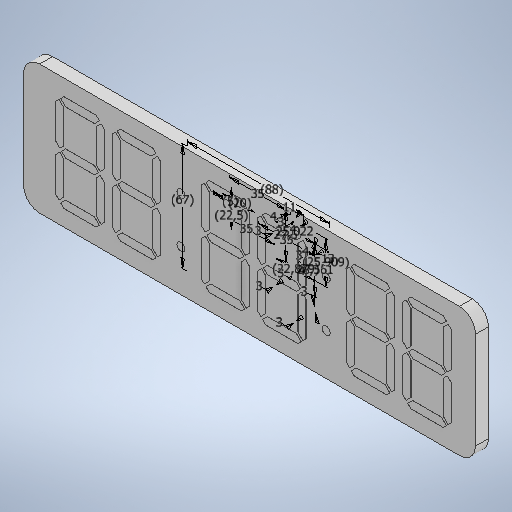
# Autodesk Inventor part: led 7 seg with sec v3
Saved by Autodesk Inventor 2026 (Build 300175000, 175)
## iProperties
Created: 2025-05-20
Part Number: led 7 seg with sec v3
Material: Generic
Document SubType Name: Modeling
Designer: Korobeynikov
Density: 1 g/cm^3
Appearance: Default
Author: Korobeynikov
Autodesk Inventor part; units mm, degrees
(part 1 of 2)
ref_plane "YZ Plane" through (0, 0, 0) normal (1, 0, 0) x (0, 1, 0)
ref_plane "XZ Plane" through (0, 0, 0) normal (0, 1, 0) x (-1, 0, 0)
ref_plane "XY Plane" through (0, 0, 0) normal (0, 0, 1) x (1, 0, 0)
sketch "Sketch1" plane through (0, 0, 0) normal (0, 0, 1) x (1, 0, 0)
  line L0 (-94.452745, 39.06468) -> (-94.589791, 54.989395)
  line L1 (-94.589791, 54.989395) -> (-92.917833, 56.661352)
  line L2 (-92.917833, 56.661352) -> (-89.738372, 53.618937)
  line L3 (-89.738372, 53.618937) -> (-89.519936, 39.107131)
  line L4 (-89.519936, 39.107131) -> (-91.876285, 36.652675)
  line L5 (-91.876285, 36.652675) -> (-94.452745, 39.06468)
  line L6 (-91.726744, 57.81642) -> (-89.962706, 59.534036)
  line L7 (-89.962706, 59.534036) -> (-75.989669, 59.62688)
  line L8 (-75.989669, 59.62688) -> (-74.318475, 57.81642)
  line L9 (-74.318475, 57.81642) -> (-77.243064, 54.845409)
  line L10 (-77.243064, 54.845409) -> (-88.659704, 54.666486)
  line L11 (-88.659704, 54.666486) -> (-91.726744, 57.81642)
  line L12 (-76.216901, 53.807549) -> (-73.431578, 57.037508)
  line L13 (-73.431578, 57.037508) -> (-71.760384, 55.412736)
  line L14 (-71.760384, 55.412736) -> (-71.161775, 39.572555)
  line L15 (-71.161775, 39.572555) -> (-73.390034, 36.97292)
  line L16 (-73.390034, 36.97292) -> (-75.989669, 39.386867)
  line L17 (-75.989669, 39.386867) -> (-76.216901, 53.807549)
  line L18 (-94.41637, 31.993238) -> (-91.950969, 34.351448)
  line L19 (-91.950969, 34.351448) -> (-89.414107, 31.993238)
  line L20 (-89.414107, 31.993238) -> (-89.235455, 17.272291)
  line L21 (-89.235455, 17.272291) -> (-92.344004, 14.02082)
  line L22 (-92.344004, 14.02082) -> (-94.41637, 15.55723)
  line L23 (-94.41637, 15.55723) -> (-94.41637, 31.993238)
  line L24 (-75.729343, 32.350542) -> (-73.442594, 34.780213)
  line L25 (-73.442594, 34.780213) -> (-71.120115, 32.350542)
  line L26 (-71.120115, 32.350542) -> (-70.584158, 16.450491)
  line L27 (-70.584158, 16.450491) -> (-72.227759, 14.449586)
  line L28 (-72.227759, 14.449586) -> (-75.47923, 17.558135)
  line L29 (-75.47923, 17.558135) -> (-75.729343, 32.350542)
  line L30 (-91.320001, 13.041828) -> (-88.199271, 16.093186)
  line L31 (-88.199271, 16.093186) -> (-76.586874, 16.486221)
  line L32 (-76.586874, 16.486221) -> (-73.478325, 13.377672)
  line L33 (-73.478325, 13.377672) -> (-75.014734, 11.62688)
  line L34 (-75.014734, 11.62688) -> (-89.360478, 11.037757)
  line L35 (-89.360478, 11.037757) -> (-91.320001, 13.041828)
  line L36 (-120.187024, 34.985074) -> (-117.790265, 37.349445)
  line L37 (-117.790265, 37.349445) -> (-105.903635, 37.640942)
  line L38 (-105.903635, 37.640942) -> (-103.442099, 35.30896)
  line L39 (-103.442099, 35.30896) -> (-106.000801, 32.847424)
  line L40 (-106.000801, 32.847424) -> (-117.806898, 32.572344)
  line L41 (-117.806898, 32.572344) -> (-120.187024, 34.985074)
  line L42 (-90.850509, 35.606243) -> (-88.45375, 37.970613)
  line L43 (-88.45375, 37.970613) -> (-76.56712, 38.262111)
  line L44 (-76.56712, 38.262111) -> (-74.105584, 35.930129)
  line L45 (-74.105584, 35.930129) -> (-76.664286, 33.468593)
  line L46 (-76.664286, 33.468593) -> (-88.470383, 33.193513)
  line L47 (-88.470383, 33.193513) -> (-90.850509, 35.606243)
  line L48 (-15, -30) -> (15, -30)
  line L49 (15, -30) -> (15, 30)
  line L50 (15, 30) -> (-15, 30)
  line L51 (-15, 30) -> (-15, -30)
  line L52 (-10, 30) -> (-10, -30)
  line L53 (10, 30) -> (10, -30)
  line L54 (-15, 25) -> (15, 25)
  line L55 (-15, -25) -> (15, -25)
  line L56 (-15, 2.5) -> (15, 2.5)
  line L57 (-15, -2.5) -> (15, -2.5)
  circle A0 centre (-12.5, 0) radius 1.06066
  line L58 (-11.43934, 0) -> (-8.93934, 2.5)
  line L59 (-11.43934, 0) -> (-8.93934, -2.5)
  line L60 (-12.5, 1.06066) -> (-15, 3.56066)
  line L61 (-12.5, 1.06066) -> (-10, 3.56066)
  line L62 (-12.5, -1.06066) -> (-15, -3.56066)
  line L63 (-12.5, -1.06066) -> (-10, -3.56066)
  line L64 (0, 8.520255) -> (0, -8.520255)
  line L65 (11.43934, 0) -> (8.93934, 2.5)
  line L66 (11.43934, 0) -> (8.93934, -2.5)
  line L67 (12.5, 1.06066) -> (15, 3.56066)
  line L68 (12.5, 1.06066) -> (10, 3.56066)
  line L69 (12.5, -1.06066) -> (15, -3.56066)
  line L70 (12.5, -1.06066) -> (10, -3.56066)
  line L71 (-15, 25) -> (-10, 30)
  line L72 (-15, 30) -> (-10, 25)
  line L73 (-13.03033, 26.96967) -> (-10, 23.93934)
  line L74 (-11.96967, 28.03033) -> (-8.93934, 25)
  line L75 (-6.230805, 0) -> (6.230805, 0)
  line L76 (13.03033, 26.96967) -> (10, 23.93934)
  line L77 (11.96967, 28.03033) -> (8.93934, 25)
  line L78 (-13.03033, -26.96967) -> (-10, -23.93934)
  line L79 (-11.96967, -28.03033) -> (-8.93934, -25)
  line L80 (13.03033, -26.96967) -> (10, -23.93934)
  line L81 (11.96967, -28.03033) -> (8.93934, -25)
  line L82 (10, 30) -> (15, 25)
  line L83 (-15, -25) -> (-10, -30)
  line L84 (10, -30) -> (15, -25)
  point P0 (0, 0)
  point P1 (-15, 0)
  point P2 (15, 0)
  point P3 (0, 0)
  dimension "d19" = 4.78147
  dimension "d20" = 48.49628
  dimension "d21" = 1.50362
  dimension "d22" = 20.00868
  dimension "d23" = 17.40827
  dimension "d24" = 22.82941
  dimension "d25" = 26.15829
  dimension "d26" = 4.82789
  dimension "d27" = 30
  dimension "d28" = 60
  dimension "d29" = 5
  dimension "d30" = 5
  dimension "d31" = 5
  dimension "d32" = 5
  dimension "d33" = 2.5
  dimension "d34" = 2.5
  dimension "d37" = 2.5
  dimension "d39" = 45
  dimension "d40" = 45
  dimension "d41" = 45
  dimension "d42" = 45
  dimension "d43" = 1.5
  dimension "d44" = 45
  dimension "d47" = 1.67119
  dimension "d50" = 0.75
  dimension "d51" = 0.75
  constraints: 168 end point, 21 symmetric about line, 17 point on line, 11 perpendicular, 3 horizontal alignment, 3 midpoint, 3 parallel, 3 point on circle, 2 horizontal, 2 vertical, 2 vertical alignment, 1 centre point, 1 coincident, 10 other
  measures "d19" vertical distance of L7.end L9.end
  measures "d20" vertical distance of L34.end L6.end
  measures "d21" distance of L10.end L2.end
  measures "d22" vertical distance of L4.end L1.end
  measures "d23" distance of L8.end L6.start
  measures "d24" horizontal distance of L13.end L0.end
  measures "d25" vertical distance of L7.end L45.end
  measures "d26" horizontal distance of L14.end L16.end
  measures "d27" distance of L50.end L49.end
  measures "d28" distance of L49.end L48.end
  measures "d30" distance between parallel lines of L49 L53
  measures "d31" distance between parallel lines of L50 L54
  measures "d32" distance between parallel lines of L48 L55
  measures "d33" distance from line of point (0, 0) L57
  measures "d34" distance from line of point (0, 0) L56
  measures "d37" distance of point (-15, 0) A0.centre
  measures "d39" angle of L57 L59
  measures "d40" angle of L56 L58
  measures "d41" angle to the sketch x axis of L60
  measures "d42" angle of L52 L61
  measures "d43" distance of L58.end L61.end
  measures "d44" angle to the sketch x axis of L62
  measures "d47" horizontal distance of L13.end L12.end
  measures "d50" distance between parallel lines of L72 L73
  measures "d51" distance between parallel lines of L74 L72
extrude "Extrusion1" add sketch "Sketch1" along normal blind 0.5 contours L52 L79 L55 L81 L53 L48 | L83 L79 L52 | L51 L62 L57 L63 L52 L78 L55 | L55 L78 L83 | L53 L81 L84 | L62 L63 L57 | L55 L80 L53 L70 L57 L69 L49 | L84 L80 L55 | L51 L54 L73 L52 L61 L56 L60 | L56 L61 L60 | L58 L52 L59 | L57 L70 L69 | L71 L73 L54 | L52 L58 L56 L64 L57 L59 | L64 L56 L65 L53 L66 L57 | L67 L56 L68 L53 L76 L54 L49 | L67 L68 L56 | L53 L65 L66 | L50 L53 L77 L54 L74 L52 | L52 L74 L71 | L54 L76 L82 | L82 L77 L53
pattern_linear "Rectangular Pattern1" count 2 spacing -35 along (-1, 0, 0) of "Extrusion1"
pattern_linear "Rectangular Pattern2" count 3 spacing 90 along (1, 0, 0) of "Extrusion1", "Rectangular Pattern1"
sketch "Sketch2" plane through (50, 3.56066, 0) normal (0, 0, -1) x (-1, 0, 0)
  line L0 (-25, 21.43934) -> (-25, 0)
  line L1 (-25, 10.71967) -> (0, 10.71967)
  line L2 (0, 0) -> (0, 21.43934)
  line L3 (-25, -7.12132) -> (-25, -28.56066)
  line L4 (-25, -17.84099) -> (0, -17.84099)
  line L5 (0, -28.56066) -> (0, -7.12132)
  circle A0 centre (-12.5, 10.71967) radius 2.5
  circle A1 centre (-12.5, -17.84099) radius 2.5
  line L6 (-115, 21.43934) -> (-115, 0)
  line L7 (-115, 10.71967) -> (-90, 10.71967)
  line L8 (-90, 0) -> (-90, 21.43934)
  line L9 (-115, -7.12132) -> (-115, -28.56066)
  line L10 (-115, -17.84099) -> (-90, -17.84099)
  line L11 (-90, -28.56066) -> (-90, -7.12132)
  circle A2 centre (-102.5, 10.71967) radius 2.5
  circle A3 centre (-102.5, -17.84099) radius 2.5
  point P0 (50, -3.56066)
  dimension "d58" = 5
  dimension "d59" = 5
  dimension "d62" = 12.5
  dimension "d203" = 5
  dimension "d204" = 5
  constraints: 12 midpoint, 8 end point, 4 centre point
  measures "d58" diameter of A0
  measures "d59" diameter of A1
  measures "d62" distance from line of L2 A0.centre
  measures "d203" diameter of A2
  measures "d204" diameter of A3
extrude "Extrusion2" add sketch "Sketch2" against normal up to surface (0.5 mm away)
sketch "Sketch3" plane through (115, 30, 0.5) normal (0, 0, 1) x (1, 0, 0)
  line L0 (-140, 10) -> (120, 10)
  line L1 (130, 0) -> (130, -60)
  line L2 (120, -70) -> (-140, -70)
  line L3 (-150, -60) -> (-150, 0)
  line L4 (25, -26.43934) -> (25, -5)
  line L5 (-130, -5) -> (-130, -26.43934)
  line L6 (-105, 0) -> (-125, 0)
  line L7 (-125, -60) -> (-105, -60)
  arc A0 (-140, 10) -> (-150, 0) centre (-140, 0) ccw
  arc A1 (-150, -60) -> (-140, -70) centre (-140, -60) ccw
  arc A2 (130, 0) -> (120, 10) centre (120, 0) ccw
  arc A3 (120, -70) -> (130, -60) centre (120, -60) ccw
  line L8 (-103.03033, -1.96967) -> (-105, 0)
  line L9 (-105, 0) -> (-125, 0)
  line L10 (-125, 0) -> (-126.96967, -1.96967)
  line L11 (-126.96967, -1.96967) -> (-123.93934, -5)
  line L12 (-123.93934, -5) -> (-106.06066, -5)
  line L13 (-106.06066, -5) -> (-103.03033, -1.96967)
  line L14 (-128.03033, -3.03033) -> (-130, -5)
  line L15 (-130, -5) -> (-130, -26.43934)
  line L16 (-130, -26.43934) -> (-127.5, -28.93934)
  line L17 (-127.5, -28.93934) -> (-125, -26.43934)
  line L18 (-125, -26.43934) -> (-125, -6.06066)
  line L19 (-125, -6.06066) -> (-128.03033, -3.03033)
  line L20 (-123.93934, -27.5) -> (-126.43934, -30)
  line L21 (-126.43934, -30) -> (-123.93934, -32.5)
  line L22 (-123.93934, -32.5) -> (-106.06066, -32.5)
  line L23 (-106.06066, -32.5) -> (-103.56066, -30)
  line L24 (-103.56066, -30) -> (-106.06066, -27.5)
  line L25 (-106.06066, -27.5) -> (-123.93934, -27.5)
  line L26 (-125, -53.93934) -> (-125, -33.56066)
  line L27 (-130, -33.56066) -> (-130, -55)
  line L28 (-125, -53.93934) -> (-125, -33.56066)
  line L29 (-125, -33.56066) -> (-127.5, -31.06066)
  line L30 (-127.5, -31.06066) -> (-130, -33.56066)
  line L31 (-130, -33.56066) -> (-130, -55)
  line L32 (-130, -55) -> (-128.03033, -56.96967)
  line L33 (-128.03033, -56.96967) -> (-125, -53.93934)
  line L34 (-106.06066, -55) -> (-123.93934, -55)
  line L35 (-106.06066, -55) -> (-123.93934, -55)
  line L36 (-123.93934, -55) -> (-126.96967, -58.03033)
  line L37 (-126.96967, -58.03033) -> (-125, -60)
  line L38 (-125, -60) -> (-105, -60)
  line L39 (-105, -60) -> (-103.03033, -58.03033)
  line L40 (-103.03033, -58.03033) -> (-106.06066, -55)
  line L41 (-101.96967, -56.96967) -> (-100, -55)
  line L42 (-100, -55) -> (-100, -33.56066)
  line L43 (-100, -33.56066) -> (-102.5, -31.06066)
  line L44 (-102.5, -31.06066) -> (-105, -33.56066)
  line L45 (-105, -33.56066) -> (-105, -53.93934)
  line L46 (-105, -53.93934) -> (-101.96967, -56.96967)
  line L47 (-105, -6.06066) -> (-105, -26.43934)
  line L48 (-105, -26.43934) -> (-102.5, -28.93934)
  line L49 (-102.5, -28.93934) -> (-100, -26.43934)
  line L50 (-100, -26.43934) -> (-100, -5)
  line L51 (-100, -5) -> (-101.96967, -3.03033)
  line L52 (-101.96967, -3.03033) -> (-105, -6.06066)
  line L53 (-90, -26.43934) -> (-90, -6.06066)
  line L54 (-93.03033, -3.03033) -> (-95, -5)
  line L55 (-95, -5) -> (-95, -26.43934)
  line L56 (-95, -26.43934) -> (-92.5, -28.93934)
  line L57 (-92.5, -28.93934) -> (-90, -26.43934)
  line L58 (-90, -26.43934) -> (-90, -6.06066)
  line L59 (-90, -6.06066) -> (-93.03033, -3.03033)
  line L60 (-68.03033, -1.96967) -> (-70, 0)
  line L61 (-70, 0) -> (-90, 0)
  line L62 (-90, 0) -> (-91.96967, -1.96967)
  line L63 (-91.96967, -1.96967) -> (-88.93934, -5)
  line L64 (-88.93934, -5) -> (-71.06066, -5)
  line L65 (-71.06066, -5) -> (-68.03033, -1.96967)
  line L66 (-70, -6.06066) -> (-70, -26.43934)
  line L67 (-70, -26.43934) -> (-67.5, -28.93934)
  line L68 (-67.5, -28.93934) -> (-65, -26.43934)
  line L69 (-65, -26.43934) -> (-65, -5)
  line L70 (-65, -5) -> (-66.96967, -3.03033)
  line L71 (-66.96967, -3.03033) -> (-70, -6.06066)
  line L72 (-88.93934, -27.5) -> (-91.43934, -30)
  line L73 (-91.43934, -30) -> (-88.93934, -32.5)
  line L74 (-88.93934, -32.5) -> (-71.06066, -32.5)
  line L75 (-71.06066, -32.5) -> (-68.56066, -30)
  line L76 (-68.56066, -30) -> (-71.06066, -27.5)
  line L77 (-71.06066, -27.5) -> (-88.93934, -27.5)
  line L78 (-95, -33.56066) -> (-95, -55)
  line L79 (-90, -53.93934) -> (-90, -33.56066)
  line L80 (-90, -33.56066) -> (-92.5, -31.06066)
  line L81 (-92.5, -31.06066) -> (-95, -33.56066)
  line L82 (-95, -33.56066) -> (-95, -55)
  line L83 (-95, -55) -> (-93.03033, -56.96967)
  line L84 (-93.03033, -56.96967) -> (-90, -53.93934)
  line L85 (-66.96967, -56.96967) -> (-65, -55)
  line L86 (-65, -55) -> (-65, -33.56066)
  line L87 (-65, -33.56066) -> (-67.5, -31.06066)
  line L88 (-67.5, -31.06066) -> (-70, -33.56066)
  line L89 (-70, -33.56066) -> (-70, -53.93934)
  line L90 (-70, -53.93934) -> (-66.96967, -56.96967)
  line L91 (-71.06066, -55) -> (-88.93934, -55)
  line L92 (-88.93934, -55) -> (-91.96967, -58.03033)
  line L93 (-91.96967, -58.03033) -> (-90, -60)
  line L94 (-90, -60) -> (-70, -60)
  line L95 (-70, -60) -> (-68.03033, -58.03033)
  line L96 (-68.03033, -58.03033) -> (-71.06066, -55)
  circle A4 centre (-52.5, -44.28033) radius 2.5
  circle A5 centre (-52.5, -15.71967) radius 2.5
  line L97 (-40, -5) -> (-40, -26.43934)
  line L98 (-13.03033, -1.96967) -> (-15, 0)
  line L99 (-15, 0) -> (-35, 0)
  line L100 (-35, 0) -> (-36.96967, -1.96967)
  line L101 (-36.96967, -1.96967) -> (-33.93934, -5)
  line L102 (-33.93934, -5) -> (-16.06066, -5)
  line L103 (-16.06066, -5) -> (-13.03033, -1.96967)
  line L104 (-15, -6.06066) -> (-15, -26.43934)
  line L105 (-15, -26.43934) -> (-12.5, -28.93934)
  line L106 (-12.5, -28.93934) -> (-10, -26.43934)
  line L107 (-10, -26.43934) -> (-10, -5)
  line L108 (-10, -5) -> (-11.96967, -3.03033)
  line L109 (-11.96967, -3.03033) -> (-15, -6.06066)
  line L110 (-38.03033, -3.03033) -> (-40, -5)
  line L111 (-40, -5) -> (-40, -26.43934)
  line L112 (-40, -26.43934) -> (-37.5, -28.93934)
  line L113 (-37.5, -28.93934) -> (-35, -26.43934)
  line L114 (-35, -26.43934) -> (-35, -6.06066)
  line L115 (-35, -6.06066) -> (-38.03033, -3.03033)
  line L116 (-33.93934, -27.5) -> (-36.43934, -30)
  line L117 (-36.43934, -30) -> (-33.93934, -32.5)
  line L118 (-33.93934, -32.5) -> (-16.06066, -32.5)
  line L119 (-16.06066, -32.5) -> (-13.56066, -30)
  line L120 (-13.56066, -30) -> (-16.06066, -27.5)
  line L121 (-16.06066, -27.5) -> (-33.93934, -27.5)
  line L122 (-35, -53.93934) -> (-35, -33.56066)
  line L123 (-35, -33.56066) -> (-37.5, -31.06066)
  line L124 (-37.5, -31.06066) -> (-40, -33.56066)
  line L125 (-40, -33.56066) -> (-40, -55)
  line L126 (-40, -55) -> (-38.03033, -56.96967)
  line L127 (-38.03033, -56.96967) -> (-35, -53.93934)
  line L128 (-16.06066, -55) -> (-33.93934, -55)
  line L129 (-33.93934, -55) -> (-36.96967, -58.03033)
  line L130 (-36.96967, -58.03033) -> (-35, -60)
  line L131 (-35, -60) -> (-15, -60)
  line L132 (-15, -60) -> (-13.03033, -58.03033)
  line L133 (-13.03033, -58.03033) -> (-16.06066, -55)
  line L134 (-11.96967, -56.96967) -> (-10, -55)
  line L135 (-10, -55) -> (-10, -33.56066)
  line L136 (-10, -33.56066) -> (-12.5, -31.06066)
  line L137 (-12.5, -31.06066) -> (-15, -33.56066)
  line L138 (-15, -33.56066) -> (-15, -53.93934)
  line L139 (-15, -53.93934) -> (-11.96967, -56.96967)
  line L140 (0, -53.93934) -> (0, -33.56066)
  line L141 (0, -33.56066) -> (-2.5, -31.06066)
  line L142 (-2.5, -31.06066) -> (-5, -33.56066)
  line L143 (-5, -33.56066) -> (-5, -55)
  line L144 (-5, -55) -> (-3.03033, -56.96967)
  line L145 (-3.03033, -56.96967) -> (0, -53.93934)
  line L146 (1.06066, -27.5) -> (-1.43934, -30)
  line L147 (-1.43934, -30) -> (1.06066, -32.5)
  line L148 (1.06066, -32.5) -> (18.93934, -32.5)
  line L149 (18.93934, -32.5) -> (21.43934, -30)
  line L150 (21.43934, -30) -> (18.93934, -27.5)
  line L151 (18.93934, -27.5) -> (1.06066, -27.5)
  line L152 (-3.03033, -3.03033) -> (-5, -5)
  line L153 (-5, -5) -> (-5, -26.43934)
  line L154 (-5, -26.43934) -> (-2.5, -28.93934)
  line L155 (-2.5, -28.93934) -> (0, -26.43934)
  line L156 (0, -26.43934) -> (0, -6.06066)
  line L157 (0, -6.06066) -> (-3.03033, -3.03033)
  line L158 (21.96967, -1.96967) -> (20, 0)
  line L159 (20, 0) -> (0, 0)
  line L160 (0, 0) -> (-1.96967, -1.96967)
  line L161 (-1.96967, -1.96967) -> (1.06066, -5)
  line L162 (1.06066, -5) -> (18.93934, -5)
  line L163 (18.93934, -5) -> (21.96967, -1.96967)
  line L164 (20, -6.06066) -> (20, -26.43934)
  line L165 (20, -26.43934) -> (22.5, -28.93934)
  line L166 (22.5, -28.93934) -> (25, -26.43934)
  line L167 (25, -26.43934) -> (25, -5)
  line L168 (25, -5) -> (23.03033, -3.03033)
  line L169 (23.03033, -3.03033) -> (20, -6.06066)
  line L170 (23.03033, -56.96967) -> (25, -55)
  line L171 (25, -55) -> (25, -33.56066)
  line L172 (25, -33.56066) -> (22.5, -31.06066)
  line L173 (22.5, -31.06066) -> (20, -33.56066)
  line L174 (20, -33.56066) -> (20, -53.93934)
  line L175 (20, -53.93934) -> (23.03033, -56.96967)
  line L176 (18.93934, -55) -> (1.06066, -55)
  line L177 (1.06066, -55) -> (-1.96967, -58.03033)
  line L178 (-1.96967, -58.03033) -> (0, -60)
  line L179 (0, -60) -> (20, -60)
  line L180 (20, -60) -> (21.96967, -58.03033)
  line L181 (21.96967, -58.03033) -> (18.93934, -55)
  line L182 (115, -26.43934) -> (115, -5)
  line L183 (111.96967, -1.96967) -> (110, 0)
  line L184 (108.93934, -5) -> (111.96967, -1.96967)
  line L185 (91.06066, -5) -> (108.93934, -5)
  line L186 (88.03033, -1.96967) -> (91.06066, -5)
  line L187 (90, 0) -> (88.03033, -1.96967)
  line L188 (110, 0) -> (90, 0)
  line L189 (110, -6.06066) -> (110, -26.43934)
  line L190 (113.03033, -3.03033) -> (110, -6.06066)
  line L191 (115, -5) -> (113.03033, -3.03033)
  line L192 (115, -26.43934) -> (115, -5)
  line L193 (112.5, -28.93934) -> (115, -26.43934)
  line L194 (110, -26.43934) -> (112.5, -28.93934)
  line L195 (113.03033, -56.96967) -> (115, -55)
  line L196 (110, -53.93934) -> (113.03033, -56.96967)
  line L197 (110, -33.56066) -> (110, -53.93934)
  line L198 (112.5, -31.06066) -> (110, -33.56066)
  line L199 (115, -33.56066) -> (112.5, -31.06066)
  line L200 (115, -55) -> (115, -33.56066)
  line L201 (91.06066, -27.5) -> (88.56066, -30)
  line L202 (108.93934, -27.5) -> (91.06066, -27.5)
  line L203 (111.43934, -30) -> (108.93934, -27.5)
  line L204 (108.93934, -32.5) -> (111.43934, -30)
  line L205 (91.06066, -32.5) -> (108.93934, -32.5)
  line L206 (88.56066, -30) -> (91.06066, -32.5)
  line L207 (90, -53.93934) -> (90, -33.56066)
  line L208 (86.96967, -56.96967) -> (90, -53.93934)
  line L209 (85, -55) -> (86.96967, -56.96967)
  line L210 (85, -33.56066) -> (85, -55)
  line L211 (87.5, -31.06066) -> (85, -33.56066)
  line L212 (90, -33.56066) -> (87.5, -31.06066)
  line L213 (108.93934, -55) -> (91.06066, -55)
  line L214 (111.96967, -58.03033) -> (108.93934, -55)
  line L215 (110, -60) -> (111.96967, -58.03033)
  line L216 (90, -60) -> (110, -60)
  line L217 (88.03033, -58.03033) -> (90, -60)
  line L218 (91.06066, -55) -> (88.03033, -58.03033)
  line L219 (86.96967, -3.03033) -> (85, -5)
  line L220 (90, -6.06066) -> (86.96967, -3.03033)
  line L221 (90, -26.43934) -> (90, -6.06066)
  line L222 (87.5, -28.93934) -> (90, -26.43934)
  line L223 (85, -26.43934) -> (87.5, -28.93934)
  line L224 (85, -5) -> (85, -26.43934)
  line L225 (76.96967, -1.96967) -> (75, 0)
  line L226 (73.93934, -5) -> (76.96967, -1.96967)
  line L227 (56.06066, -5) -> (73.93934, -5)
  line L228 (53.03033, -1.96967) -> (56.06066, -5)
  line L229 (55, 0) -> (53.03033, -1.96967)
  line L230 (75, 0) -> (55, 0)
  line L231 (75, -6.06066) -> (75, -26.43934)
  line L232 (78.03033, -3.03033) -> (75, -6.06066)
  line L233 (80, -5) -> (78.03033, -3.03033)
  line L234 (80, -26.43934) -> (80, -5)
  line L235 (77.5, -28.93934) -> (80, -26.43934)
  line L236 (75, -26.43934) -> (77.5, -28.93934)
  line L237 (56.06066, -27.5) -> (53.56066, -30)
  line L238 (73.93934, -27.5) -> (56.06066, -27.5)
  line L239 (76.43934, -30) -> (73.93934, -27.5)
  line L240 (73.93934, -32.5) -> (76.43934, -30)
  line L241 (56.06066, -32.5) -> (73.93934, -32.5)
  line L242 (53.56066, -30) -> (56.06066, -32.5)
  line L243 (78.03033, -56.96967) -> (80, -55)
  line L244 (75, -53.93934) -> (78.03033, -56.96967)
  line L245 (75, -33.56066) -> (75, -53.93934)
  line L246 (77.5, -31.06066) -> (75, -33.56066)
  line L247 (80, -33.56066) -> (77.5, -31.06066)
  line L248 (80, -55) -> (80, -33.56066)
  line L249 (73.93934, -55) -> (56.06066, -55)
  line L250 (76.96967, -58.03033) -> (73.93934, -55)
  line L251 (75, -60) -> (76.96967, -58.03033)
  line L252 (55, -60) -> (75, -60)
  line L253 (53.03033, -58.03033) -> (55, -60)
  line L254 (56.06066, -55) -> (53.03033, -58.03033)
  line L255 (55, -53.93934) -> (55, -33.56066)
  line L256 (51.96967, -56.96967) -> (55, -53.93934)
  line L257 (50, -55) -> (51.96967, -56.96967)
  line L258 (50, -33.56066) -> (50, -55)
  line L259 (52.5, -31.06066) -> (50, -33.56066)
  line L260 (55, -33.56066) -> (52.5, -31.06066)
  line L261 (51.96967, -3.03033) -> (50, -5)
  line L262 (55, -6.06066) -> (51.96967, -3.03033)
  line L263 (55, -26.43934) -> (55, -6.06066)
  line L264 (52.5, -28.93934) -> (55, -26.43934)
  line L265 (50, -26.43934) -> (52.5, -28.93934)
  line L266 (50, -5) -> (50, -26.43934)
  circle A6 centre (37.5, -44.28033) radius 2.5
  circle A7 centre (37.5, -15.71967) radius 2.5
  point P0 (-115, -30)
  dimension "d64" = 20
  dimension "d65" = 10
  dimension "d66" = 10
  dimension "d67" = 10
  dimension "d68" = 10
  dimension "d205" = 15
  dimension "d206" = 280
  constraints: 8 end point, 8 point on circle, 8 tangent, 4 centre point, 2 equal radius, 2 parallel, 1 horizontal, 1 perpendicular
  measures "d64" distance between parallel lines of L3 L5
  measures "d65" distance between parallel lines of L6 L0
  measures "d66" distance between parallel lines of L2 L7
  measures "d67" radius of A0
  measures "d68" radius of A1
  measures "d205" distance between parallel lines of L1 L182
  measures "d206" distance between parallel lines of L3 L1
extrude "Extrusion3" add sketch "Sketch3" along normal blind 0.05 and the other way blind 8
sketch "Sketch4" plane through (115, 30, -7.5) normal (0, 0, -1) x (-1, 0, 0)
  line L0 (-120, -70) -> (140, -70)
  arc A0 (140, -70) -> (150, -60) centre (140, -60) ccw
  line L1 (150, -60) -> (150, 0)
  arc A1 (150, 0) -> (140, 10) centre (140, 0) ccw
  line L2 (140, 10) -> (-120, 10)
  arc A2 (-120, 10) -> (-130, 0) centre (-120, 0) ccw
  line L3 (-130, 0) -> (-130, -60)
  arc A3 (-130, -60) -> (-120, -70) centre (-120, -60) ccw
  circle A4 centre (52.5, -15.71967) radius 2.5
  line L4 (-22.5, -28.93934) -> (-25, -26.43934)
  line L5 (-25, -26.43934) -> (-25, -5)
  line L6 (-25, -5) -> (-23.03033, -3.03033)
  line L7 (-23.03033, -3.03033) -> (-20, -6.06066)
  line L8 (-20, -6.06066) -> (-20, -26.43934)
  line L9 (-20, -26.43934) -> (-22.5, -28.93934)
  line L10 (128.03033, -3.03033) -> (130, -5)
  line L11 (130, -5) -> (130, -26.43934)
  line L12 (130, -26.43934) -> (127.5, -28.93934)
  line L13 (127.5, -28.93934) -> (125, -26.43934)
  line L14 (125, -26.43934) -> (125, -6.06066)
  line L15 (125, -6.06066) -> (128.03033, -3.03033)
  line L16 (103.03033, -1.96967) -> (105, 0)
  line L17 (105, 0) -> (125, 0)
  line L18 (125, 0) -> (126.96967, -1.96967)
  line L19 (126.96967, -1.96967) -> (123.93934, -5)
  line L20 (123.93934, -5) -> (106.06066, -5)
  line L21 (106.06066, -5) -> (103.03033, -1.96967)
  line L22 (126.96967, -58.03033) -> (125, -60)
  line L23 (125, -60) -> (105, -60)
  line L24 (105, -60) -> (103.03033, -58.03033)
  line L25 (103.03033, -58.03033) -> (106.06066, -55)
  line L26 (106.06066, -55) -> (123.93934, -55)
  line L27 (123.93934, -55) -> (126.96967, -58.03033)
  line L28 (127.5, -31.06066) -> (130, -33.56066)
  line L29 (130, -33.56066) -> (130, -55)
  line L30 (130, -55) -> (128.03033, -56.96967)
  line L31 (128.03033, -56.96967) -> (125, -53.93934)
  line L32 (125, -53.93934) -> (125, -33.56066)
  line L33 (125, -33.56066) -> (127.5, -31.06066)
  line L34 (92.5, -28.93934) -> (90, -26.43934)
  line L35 (90, -26.43934) -> (90, -6.06066)
  line L36 (90, -6.06066) -> (93.03033, -3.03033)
  line L37 (93.03033, -3.03033) -> (95, -5)
  line L38 (95, -5) -> (95, -26.43934)
  line L39 (95, -26.43934) -> (92.5, -28.93934)
  line L40 (92.5, -31.06066) -> (95, -33.56066)
  line L41 (95, -33.56066) -> (95, -55)
  line L42 (95, -55) -> (93.03033, -56.96967)
  line L43 (93.03033, -56.96967) -> (90, -53.93934)
  line L44 (90, -53.93934) -> (90, -33.56066)
  line L45 (90, -33.56066) -> (92.5, -31.06066)
  circle A5 centre (52.5, -44.28033) radius 2.5
  line L46 (38.03033, -3.03033) -> (40, -5)
  line L47 (40, -5) -> (40, -26.43934)
  line L48 (40, -26.43934) -> (37.5, -28.93934)
  line L49 (37.5, -28.93934) -> (35, -26.43934)
  line L50 (35, -26.43934) -> (35, -6.06066)
  line L51 (35, -6.06066) -> (38.03033, -3.03033)
  line L52 (-21.96967, -58.03033) -> (-18.93934, -55)
  line L53 (-18.93934, -55) -> (-1.06066, -55)
  line L54 (-1.06066, -55) -> (1.96967, -58.03033)
  line L55 (1.96967, -58.03033) -> (0, -60)
  line L56 (0, -60) -> (-20, -60)
  line L57 (-20, -60) -> (-21.96967, -58.03033)
  line L58 (-20, -53.93934) -> (-23.03033, -56.96967)
  line L59 (-23.03033, -56.96967) -> (-25, -55)
  line L60 (-25, -55) -> (-25, -33.56066)
  line L61 (-25, -33.56066) -> (-22.5, -31.06066)
  line L62 (-22.5, -31.06066) -> (-20, -33.56066)
  line L63 (-20, -33.56066) -> (-20, -53.93934)
  line L64 (-18.93934, -5) -> (-21.96967, -1.96967)
  line L65 (-21.96967, -1.96967) -> (-20, 0)
  line L66 (-20, 0) -> (0, 0)
  line L67 (0, 0) -> (1.96967, -1.96967)
  line L68 (1.96967, -1.96967) -> (-1.06066, -5)
  line L69 (-1.06066, -5) -> (-18.93934, -5)
  line L70 (0, -6.06066) -> (3.03033, -3.03033)
  line L71 (3.03033, -3.03033) -> (5, -5)
  line L72 (5, -5) -> (5, -26.43934)
  line L73 (5, -26.43934) -> (2.5, -28.93934)
  line L74 (2.5, -28.93934) -> (0, -26.43934)
  line L75 (0, -26.43934) -> (0, -6.06066)
  line L76 (-18.93934, -27.5) -> (-1.06066, -27.5)
  line L77 (-1.06066, -27.5) -> (1.43934, -30)
  line L78 (1.43934, -30) -> (-1.06066, -32.5)
  line L79 (-1.06066, -32.5) -> (-18.93934, -32.5)
  line L80 (-18.93934, -32.5) -> (-21.43934, -30)
  line L81 (-21.43934, -30) -> (-18.93934, -27.5)
  line L82 (3.03033, -56.96967) -> (0, -53.93934)
  line L83 (0, -53.93934) -> (0, -33.56066)
  line L84 (0, -33.56066) -> (2.5, -31.06066)
  line L85 (2.5, -31.06066) -> (5, -33.56066)
  line L86 (5, -33.56066) -> (5, -55)
  line L87 (5, -55) -> (3.03033, -56.96967)
  line L88 (15, -53.93934) -> (11.96967, -56.96967)
  line L89 (11.96967, -56.96967) -> (10, -55)
  line L90 (10, -55) -> (10, -33.56066)
  line L91 (10, -33.56066) -> (12.5, -31.06066)
  line L92 (12.5, -31.06066) -> (15, -33.56066)
  line L93 (15, -33.56066) -> (15, -53.93934)
  line L94 (13.03033, -58.03033) -> (16.06066, -55)
  line L95 (16.06066, -55) -> (33.93934, -55)
  line L96 (33.93934, -55) -> (36.96967, -58.03033)
  line L97 (36.96967, -58.03033) -> (35, -60)
  line L98 (35, -60) -> (15, -60)
  line L99 (15, -60) -> (13.03033, -58.03033)
  line L100 (38.03033, -56.96967) -> (35, -53.93934)
  line L101 (35, -53.93934) -> (35, -33.56066)
  line L102 (35, -33.56066) -> (37.5, -31.06066)
  line L103 (37.5, -31.06066) -> (40, -33.56066)
  line L104 (40, -33.56066) -> (40, -55)
  line L105 (40, -55) -> (38.03033, -56.96967)
  line L106 (16.06066, -27.5) -> (33.93934, -27.5)
  line L107 (33.93934, -27.5) -> (36.43934, -30)
  line L108 (36.43934, -30) -> (33.93934, -32.5)
  line L109 (33.93934, -32.5) -> (16.06066, -32.5)
  line L110 (16.06066, -32.5) -> (13.56066, -30)
  line L111 (13.56066, -30) -> (16.06066, -27.5)
  line L112 (11.96967, -3.03033) -> (15, -6.06066)
  line L113 (15, -6.06066) -> (15, -26.43934)
  line L114 (15, -26.43934) -> (12.5, -28.93934)
  line L115 (12.5, -28.93934) -> (10, -26.43934)
  line L116 (10, -26.43934) -> (10, -5)
  line L117 (10, -5) -> (11.96967, -3.03033)
  line L118 (16.06066, -5) -> (13.03033, -1.96967)
  line L119 (13.03033, -1.96967) -> (15, 0)
  line L120 (15, 0) -> (35, 0)
  line L121 (35, 0) -> (36.96967, -1.96967)
  line L122 (36.96967, -1.96967) -> (33.93934, -5)
  line L123 (33.93934, -5) -> (16.06066, -5)
  line L124 (68.03033, -58.03033) -> (71.06066, -55)
  line L125 (71.06066, -55) -> (88.93934, -55)
  line L126 (88.93934, -55) -> (91.96967, -58.03033)
  line L127 (91.96967, -58.03033) -> (90, -60)
  line L128 (90, -60) -> (70, -60)
  line L129 (70, -60) -> (68.03033, -58.03033)
  line L130 (70, -53.93934) -> (66.96967, -56.96967)
  line L131 (66.96967, -56.96967) -> (65, -55)
  line L132 (65, -55) -> (65, -33.56066)
  line L133 (65, -33.56066) -> (67.5, -31.06066)
  line L134 (67.5, -31.06066) -> (70, -33.56066)
  line L135 (70, -33.56066) -> (70, -53.93934)
  line L136 (71.06066, -27.5) -> (88.93934, -27.5)
  line L137 (88.93934, -27.5) -> (91.43934, -30)
  line L138 (91.43934, -30) -> (88.93934, -32.5)
  line L139 (88.93934, -32.5) -> (71.06066, -32.5)
  line L140 (71.06066, -32.5) -> (68.56066, -30)
  line L141 (68.56066, -30) -> (71.06066, -27.5)
  line L142 (66.96967, -3.03033) -> (70, -6.06066)
  line L143 (70, -6.06066) -> (70, -26.43934)
  line L144 (70, -26.43934) -> (67.5, -28.93934)
  line L145 (67.5, -28.93934) -> (65, -26.43934)
  line L146 (65, -26.43934) -> (65, -5)
  line L147 (65, -5) -> (66.96967, -3.03033)
  line L148 (71.06066, -5) -> (68.03033, -1.96967)
  line L149 (68.03033, -1.96967) -> (70, 0)
  line L150 (70, 0) -> (90, 0)
  line L151 (90, 0) -> (91.96967, -1.96967)
  line L152 (91.96967, -1.96967) -> (88.93934, -5)
  line L153 (88.93934, -5) -> (71.06066, -5)
  line L154 (101.96967, -3.03033) -> (105, -6.06066)
  line L155 (105, -6.06066) -> (105, -26.43934)
  line L156 (105, -26.43934) -> (102.5, -28.93934)
  line L157 (102.5, -28.93934) -> (100, -26.43934)
  line L158 (100, -26.43934) -> (100, -5)
  line L159 (100, -5) -> (101.96967, -3.03033)
  line L160 (105, -53.93934) -> (101.96967, -56.96967)
  line L161 (101.96967, -56.96967) -> (100, -55)
  line L162 (100, -55) -> (100, -33.56066)
  line L163 (100, -33.56066) -> (102.5, -31.06066)
  line L164 (102.5, -31.06066) -> (105, -33.56066)
  line L165 (105, -33.56066) -> (105, -53.93934)
  line L166 (106.06066, -27.5) -> (123.93934, -27.5)
  line L167 (123.93934, -27.5) -> (126.43934, -30)
  line L168 (126.43934, -30) -> (123.93934, -32.5)
  line L169 (123.93934, -32.5) -> (106.06066, -32.5)
  line L170 (106.06066, -32.5) -> (103.56066, -30)
  line L171 (103.56066, -30) -> (106.06066, -27.5)
  line L172 (-120, 8) -> (140, 8)
  arc A6 (148, 0) -> (140, 8) centre (140, 0) ccw
  line L173 (148, 0) -> (148, -60)
  arc A7 (140, -68) -> (148, -60) centre (140, -60) ccw
  line L174 (140, -68) -> (-120, -68)
  arc A8 (-128, -60) -> (-120, -68) centre (-120, -60) ccw
  line L175 (-128, -60) -> (-128, 0)
  arc A9 (-120, 8) -> (-128, 0) centre (-120, 0) ccw
  line L176 (-20, -5) -> (0, -5)
  line L177 (0, -5) -> (0, -27.5)
  line L178 (0, -27.5) -> (-20, -27.5)
  line L179 (-20, -27.5) -> (-20, -5)
  line L180 (-20, -32.5) -> (0, -32.5)
  line L181 (0, -32.5) -> (0, -55)
  line L182 (0, -55) -> (-20, -55)
  line L183 (-20, -55) -> (-20, -32.5)
  line L184 (-18.5, -6.5) -> (-1.5, -6.5)
  line L185 (-1.5, -6.5) -> (-1.5, -26)
  line L186 (-1.5, -26) -> (-18.5, -26)
  line L187 (-18.5, -26) -> (-18.5, -6.5)
  line L188 (-1.5, -34) -> (-18.5, -34)
  line L189 (-18.5, -34) -> (-18.5, -53.5)
  line L190 (-18.5, -53.5) -> (-1.5, -53.5)
  line L191 (-1.5, -53.5) -> (-1.5, -34)
  line L192 (16.5, -6.5) -> (33.5, -6.5)
  line L193 (16.5, -26) -> (16.5, -6.5)
  line L194 (33.5, -6.5) -> (33.5, -26)
  line L195 (33.5, -26) -> (16.5, -26)
  line L196 (33.5, -34) -> (16.5, -34)
  line L197 (16.5, -34) -> (16.5, -53.5)
  line L198 (33.5, -53.5) -> (33.5, -34)
  line L199 (16.5, -53.5) -> (33.5, -53.5)
  line L200 (71.5, -26) -> (71.5, -6.5)
  line L201 (71.5, -6.5) -> (88.5, -6.5)
  line L202 (88.5, -6.5) -> (88.5, -26)
  line L203 (88.5, -26) -> (71.5, -26)
  line L204 (88.5, -34) -> (71.5, -34)
  line L205 (71.5, -34) -> (71.5, -53.5)
  line L206 (88.5, -53.5) -> (88.5, -34)
  line L207 (71.5, -53.5) -> (88.5, -53.5)
  line L208 (106.5, -26) -> (106.5, -6.5)
  line L209 (106.5, -6.5) -> (123.5, -6.5)
  line L210 (123.5, -6.5) -> (123.5, -26)
  line L211 (123.5, -26) -> (106.5, -26)
  line L212 (123.5, -34) -> (106.5, -34)
  line L213 (123.5, -53.5) -> (123.5, -34)
  line L214 (106.5, -34) -> (106.5, -53.5)
  line L215 (106.5, -53.5) -> (123.5, -53.5)
  line L216 (-25, 0) -> (40, 0)
  line L217 (40, 0) -> (40, -60)
  line L218 (40, -60) -> (-25, -60)
  line L219 (-25, -60) -> (-25, 0)
  line L220 (41.5, 1.5) -> (-26.5, 1.5)
  line L221 (-26.5, 1.5) -> (-26.5, -61.5)
  line L222 (-26.5, -61.5) -> (41.5, -61.5)
  line L223 (41.5, -61.5) -> (41.5, 1.5)
  line L224 (131.5, 1.5) -> (63.5, 1.5)
  line L225 (63.5, 1.5) -> (63.5, -61.5)
  line L226 (131.5, -61.5) -> (131.5, 1.5)
  line L227 (63.5, -61.5) -> (131.5, -61.5)
  circle A10 centre (52.5, -15.71967) radius 4
  circle A11 centre (52.5, -44.28033) radius 4
  line L228 (-48.5, 1.5) -> (-116.5, 1.5)
  line L229 (-48.5, -61.5) -> (-48.5, 1.5)
  line L230 (-116.5, -61.5) -> (-48.5, -61.5)
  line L231 (-116.5, 1.5) -> (-116.5, -61.5)
  line L232 (-108.5, -26) -> (-108.5, -6.5)
  line L233 (-108.5, -6.5) -> (-91.5, -6.5)
  line L234 (-91.5, -6.5) -> (-91.5, -26)
  line L235 (-91.5, -26) -> (-108.5, -26)
  line L236 (-91.5, -34) -> (-108.5, -34)
  line L237 (-108.5, -34) -> (-108.5, -53.5)
  line L238 (-108.5, -53.5) -> (-91.5, -53.5)
  line L239 (-91.5, -53.5) -> (-91.5, -34)
  line L240 (-73.5, -34) -> (-73.5, -53.5)
  line L241 (-56.5, -34) -> (-73.5, -34)
  line L242 (-73.5, -26) -> (-73.5, -6.5)
  line L243 (-56.5, -26) -> (-73.5, -26)
  line L244 (-73.5, -6.5) -> (-56.5, -6.5)
  line L245 (-56.5, -6.5) -> (-56.5, -26)
  line L246 (-56.5, -53.5) -> (-56.5, -34)
  line L247 (-73.5, -53.5) -> (-56.5, -53.5)
  circle A12 centre (-37.5, -15.71967) radius 2.5
  circle A13 centre (-37.5, -15.71967) radius 4
  circle A14 centre (-37.5, -44.28033) radius 2.5
  circle A15 centre (-37.5, -44.28033) radius 4
  point P0 (115, -30)
  dimension "d73" = 2
  dimension "d75" = 1.5
  dimension "d76" = 1.5
  dimension "d79" = 35
  dimension "d86" = 90
  dimension "d92" = 1.5
  dimension "d95" = 90
  dimension "d100" = 1.5
  dimension "d101" = 1.5
  dimension "d216" = 90
  constraints: 152 end point, 12 parallel, 8 centre point, 8 point on circle, 7 horizontal, 6 perpendicular, 3 collinear, 3 point on line, 2 coincident, 2 equal radius, 109 other
  measures "d73" distance between parallel lines of L2 L172
  measures "d75" distance between parallel lines of L179 L187
  measures "d76" distance between parallel lines of L180 L188
  measures "d79" distance of L184.start L192.start
  measures "d86" distance of L186.end L200.start
  measures "d92" distance between parallel lines of L216 L220
  measures "d95" distance of L220.start L224.start
  measures "d100" radial gap between concentric circles of A4 A10
  measures "d101" radial gap between concentric circles of A5 A11
  measures "d216" distance of L220.start L228.start
extrude "Extrusion4" cut sketch "Sketch4" against normal blind 7 contours L172 A6 L173 A7 L174 A8 L175 A9 | L184 L185 L186 L187 | L191 L190 L189 L188 | L192 L194 L195 L193 | L198 L199 L197 L196 | L200 L201 L202 L203 | L206 L207 L205 L204 | L208 L209 L210 L211 | L213 L215 L214 L212 | L232 L233 L234 L235 | L239 L238 L237 L236 | L241 L246 L247 L240 | L242 L244 L245 L243 | A12 | A14
sketch "Sketch5" plane through (115, 30, -7.5) normal (0, 0, -1) x (-1, 0, 0)
  line L0 (-1.5, -53.5) -> (-18.5, -53.5)
  line L1 (-18.5, -53.5) -> (-18.5, -34)
  line L2 (-18.5, -34) -> (-1.5, -34)
  line L3 (-1.5, -34) -> (-1.5, -53.5)
  line L4 (33.5, -53.5) -> (16.5, -53.5)
  line L5 (16.5, -53.5) -> (16.5, -34)
  line L6 (16.5, -34) -> (33.5, -34)
  line L7 (33.5, -34) -> (33.5, -53.5)
  line L8 (-1.5, -6.5) -> (-1.5, -26)
  line L9 (-1.5, -26) -> (-18.5, -26)
  line L10 (-18.5, -26) -> (-18.5, -6.5)
  line L11 (-18.5, -6.5) -> (-1.5, -6.5)
  line L12 (33.5, -6.5) -> (33.5, -26)
  line L13 (33.5, -26) -> (16.5, -26)
  line L14 (16.5, -26) -> (16.5, -6.5)
  line L15 (16.5, -6.5) -> (33.5, -6.5)
  line L16 (-26.5, -61.5) -> (41.5, -61.5)
  line L17 (41.5, -61.5) -> (41.5, 1.5)
  line L18 (41.5, 1.5) -> (-26.5, 1.5)
  line L19 (-26.5, 1.5) -> (-26.5, -61.5)
  line L20 (-22.5, -28.93934) -> (-25, -26.43934)
  line L21 (-25, -26.43934) -> (-25, -5)
  line L22 (-25, -5) -> (-23.03033, -3.03033)
  line L23 (-23.03033, -3.03033) -> (-20, -6.06066)
  line L24 (-20, -6.06066) -> (-20, -26.43934)
  line L25 (-20, -26.43934) -> (-22.5, -28.93934)
  line L26 (38.03033, -3.03033) -> (40, -5)
  line L27 (40, -5) -> (40, -26.43934)
  line L28 (40, -26.43934) -> (37.5, -28.93934)
  line L29 (37.5, -28.93934) -> (35, -26.43934)
  line L30 (35, -26.43934) -> (35, -6.06066)
  line L31 (35, -6.06066) -> (38.03033, -3.03033)
  line L32 (-21.96967, -58.03033) -> (-18.93934, -55)
  line L33 (-18.93934, -55) -> (-1.06066, -55)
  line L34 (-1.06066, -55) -> (1.96967, -58.03033)
  line L35 (1.96967, -58.03033) -> (0, -60)
  line L36 (0, -60) -> (-20, -60)
  line L37 (-20, -60) -> (-21.96967, -58.03033)
  line L38 (-20, -53.93934) -> (-23.03033, -56.96967)
  line L39 (-23.03033, -56.96967) -> (-25, -55)
  line L40 (-25, -55) -> (-25, -33.56066)
  line L41 (-25, -33.56066) -> (-22.5, -31.06066)
  line L42 (-22.5, -31.06066) -> (-20, -33.56066)
  line L43 (-20, -33.56066) -> (-20, -53.93934)
  line L44 (-18.93934, -5) -> (-21.96967, -1.96967)
  line L45 (-21.96967, -1.96967) -> (-20, 0)
  line L46 (-20, 0) -> (0, 0)
  line L47 (0, 0) -> (1.96967, -1.96967)
  line L48 (1.96967, -1.96967) -> (-1.06066, -5)
  line L49 (-1.06066, -5) -> (-18.93934, -5)
  line L50 (0, -6.06066) -> (3.03033, -3.03033)
  line L51 (3.03033, -3.03033) -> (5, -5)
  line L52 (5, -5) -> (5, -26.43934)
  line L53 (5, -26.43934) -> (2.5, -28.93934)
  line L54 (2.5, -28.93934) -> (0, -26.43934)
  line L55 (0, -26.43934) -> (0, -6.06066)
  line L56 (-18.93934, -27.5) -> (-1.06066, -27.5)
  line L57 (-1.06066, -27.5) -> (1.43934, -30)
  line L58 (1.43934, -30) -> (-1.06066, -32.5)
  line L59 (-1.06066, -32.5) -> (-18.93934, -32.5)
  line L60 (-18.93934, -32.5) -> (-21.43934, -30)
  line L61 (-21.43934, -30) -> (-18.93934, -27.5)
  line L62 (3.03033, -56.96967) -> (0, -53.93934)
  line L63 (0, -53.93934) -> (0, -33.56066)
  line L64 (0, -33.56066) -> (2.5, -31.06066)
  line L65 (2.5, -31.06066) -> (5, -33.56066)
  line L66 (5, -33.56066) -> (5, -55)
  line L67 (5, -55) -> (3.03033, -56.96967)
  line L68 (15, -53.93934) -> (11.96967, -56.96967)
  line L69 (11.96967, -56.96967) -> (10, -55)
  line L70 (10, -55) -> (10, -33.56066)
  line L71 (10, -33.56066) -> (12.5, -31.06066)
  line L72 (12.5, -31.06066) -> (15, -33.56066)
  line L73 (15, -33.56066) -> (15, -53.93934)
  line L74 (13.03033, -58.03033) -> (16.06066, -55)
  line L75 (16.06066, -55) -> (33.93934, -55)
  line L76 (33.93934, -55) -> (36.96967, -58.03033)
  line L77 (36.96967, -58.03033) -> (35, -60)
  line L78 (35, -60) -> (15, -60)
  line L79 (15, -60) -> (13.03033, -58.03033)
  line L80 (38.03033, -56.96967) -> (35, -53.93934)
  line L81 (35, -53.93934) -> (35, -33.56066)
  line L82 (35, -33.56066) -> (37.5, -31.06066)
  line L83 (37.5, -31.06066) -> (40, -33.56066)
  line L84 (40, -33.56066) -> (40, -55)
  line L85 (40, -55) -> (38.03033, -56.96967)
  line L86 (16.06066, -27.5) -> (33.93934, -27.5)
  line L87 (33.93934, -27.5) -> (36.43934, -30)
  line L88 (36.43934, -30) -> (33.93934, -32.5)
  line L89 (33.93934, -32.5) -> (16.06066, -32.5)
  line L90 (16.06066, -32.5) -> (13.56066, -30)
  line L91 (13.56066, -30) -> (16.06066, -27.5)
  line L92 (11.96967, -3.03033) -> (15, -6.06066)
  line L93 (15, -6.06066) -> (15, -26.43934)
  line L94 (15, -26.43934) -> (12.5, -28.93934)
  line L95 (12.5, -28.93934) -> (10, -26.43934)
  line L96 (10, -26.43934) -> (10, -5)
  line L97 (10, -5) -> (11.96967, -3.03033)
  line L98 (16.06066, -5) -> (13.03033, -1.96967)
  line L99 (13.03033, -1.96967) -> (15, 0)
  line L100 (15, 0) -> (35, 0)
  line L101 (35, 0) -> (36.96967, -1.96967)
  line L102 (36.96967, -1.96967) -> (33.93934, -5)
  line L103 (33.93934, -5) -> (16.06066, -5)
  circle A0 centre (52.5, -15.71967) radius 4
  circle A1 centre (52.5, -15.71967) radius 2.5
  circle A2 centre (52.5, -44.28033) radius 2.5
  circle A3 centre (52.5, -44.28033) radius 4
  line L104 (148, 0) -> (148, -60)
  line L105 (131.5, -61.5) -> (131.5, 1.5)
  line L106 (63.5, 1.5) -> (63.5, -61.5)
  line L107 (150, -60) -> (150, 0)
  line L108 (-130, 0) -> (-130, -60)
  line L109 (-31.5, 3.5) -> (56.5, 3.5)
  line L110 (56.5, 3.5) -> (56.5, -63.5)
  line L111 (56.5, -63.5) -> (-31.5, -63.5)
  line L112 (-31.5, -63.5) -> (-31.5, 3.5)
  circle A4 centre (52.5, -0.5) radius 2.15
  circle A5 centre (52.5, -0.5) radius 4
  circle A6 centre (-27.5, -0.5) radius 4
  circle A7 centre (-27.5, -0.5) radius 2.15
  circle A8 centre (52.5, -59.5) radius 4
  circle A9 centre (52.5, -59.5) radius 2.15
  circle A10 centre (-27.5, -59.5) radius 4
  circle A11 centre (-27.5, -59.5) radius 2.15
  circle A12 centre (62.5, -0.5) radius 4
  circle A13 centre (62.5, -0.5) radius 2.15
  line L113 (58.5, 3.5) -> (146.5, 3.5)
  circle A14 centre (142.5, -0.5) radius 4
  circle A15 centre (142.5, -0.5) radius 2.15
  line L114 (146.5, 3.5) -> (146.5, -63.5)
  circle A16 centre (142.5, -59.5) radius 4
  circle A17 centre (142.5, -59.5) radius 2.15
  line L115 (146.5, -63.5) -> (58.5, -63.5)
  circle A18 centre (62.5, -59.5) radius 4
  circle A19 centre (62.5, -59.5) radius 2.15
  line L116 (58.5, -63.5) -> (58.5, 3.5)
  line L117 (-121.5, 3.5) -> (-33.5, 3.5)
  line L118 (-121.5, -63.5) -> (-121.5, 3.5)
  line L119 (-33.5, 3.5) -> (-33.5, -63.5)
  line L120 (-33.5, -63.5) -> (-121.5, -63.5)
  circle A20 centre (-117.5, -59.5) radius 4
  circle A21 centre (-117.5, -59.5) radius 2.15
  circle A22 centre (-117.5, -0.5) radius 4
  circle A23 centre (-117.5, -0.5) radius 2.15
  circle A24 centre (-37.5, -0.5) radius 4
  circle A25 centre (-37.5, -0.5) radius 2.15
  circle A26 centre (-37.5, -59.5) radius 4
  circle A27 centre (-37.5, -59.5) radius 2.15
  point P0 (115, -30)
  point P1 (-1.5, -16.25)
  point P2 (56.5, -30.71967)
  point P3 (-26.5, -30)
  point P4 (-31.5, -30)
  point P5 (58.5, -30)
  point P6 (63.5, 1.403287)
  point P7 (63.5, -2.403287)
  point P8 (63.5, -57.596713)
  point P9 (63.5, -61.403287)
  point P10 (-26.5, -57.596713)
  point P11 (-26.5, -61.403287)
  point P12 (-26.5, 1.403287)
  point P13 (-26.5, -2.403287)
  point P14 (-121.5, -30)
  dimension "d104" = 68
  dimension "d105" = 63
  dimension "d107" = 17
  dimension "d108" = 19.5
  dimension "d109" = 15
  dimension "d110" = 16.5
  dimension "d112" = 280
  dimension "d114" = 7
  dimension "d115" = 5
  dimension "d116" = 67
  dimension "d117" = 88
  dimension "bobyshka_d" = 4.3
  dimension "d119" = 8
  dimension "d120" = 8
  dimension "d121" = 4.3
  dimension "d122" = 8
  dimension "d123" = 4.3
  dimension "d124" = 8
  dimension "d125" = 4.3
  dimension "d128" = 90
  dimension "d209" = 90
  constraints: 24 centre point, 24 end point, 12 coincident, 9 tangent, 3 horizontal, 3 midpoint, 2 collinear, 2 parallel, 1 horizontal alignment, 1 perpendicular, 48 other
  measures "d104" distance between parallel lines of L17 L19
  measures "d105" distance of L18.end L16.start
  measures "d107" distance from line of point (-1.5, -16.25) L10
  measures "d108" distance between parallel lines of L9 L11
  measures "d109" distance from line of point (56.5, -30.72) L17
  measures "d110" distance between parallel lines of L104 L105
  measures "d112" distance between parallel lines of L107 L108
  measures "d114" distance between parallel lines of L106 L110
  measures "d115" distance between parallel lines of L112 L19
  measures "d116" distance of L111.end L109.start
  measures "d117" distance of L109.start L109.end
  measures "bobyshka_d" diameter of A4
  measures "d119" diameter of A5
  measures "d120" diameter of A6
  measures "d121" diameter of A7
  measures "d122" diameter of A8
  measures "d123" diameter of A9
  measures "d124" diameter of A10
  measures "d125" diameter of A11
  measures "d128" distance of A6.centre A12.centre
  measures "d209" distance of L109.start L117.start
extrude "Extrusion5" add sketch "Sketch5" against normal up to surface (7 mm away) contours L19 A11 A10 L16 | L16 A10 L19 A11 | A8 | A6 L19 A7 L18 | L18 L19 A7 A6 | A5 | A12 | A18 | A14 | A16 | A22 | A24 | A20 | A26
extrude "Extrusion6" cut sketch "Sketch5" against normal up to surface (7 mm away) contours L19 A11 | L19 A7 | A13 L106 | A19 L106 | A21 | A23 picked at (-26.116667, -59.5) picked at (-26.116667, -0.5) picked at (64.102693, -0.455136) picked at (64.102693, -59.455136)